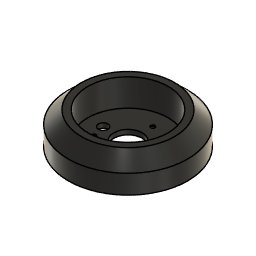
knobFlangeRev v5 (Autodesk Fusion 360 design; units mm, degrees)
Autodesk Fusion 360 part; units mm, degrees
note: some values were not read from the file. Chosen so that the rebuilt part matches the saved one: which face or edge a step refers to.
sketch "Sketch11" plane through (0, 0, 0) normal (0, 0, 1) x (1, 0, 0)
  circle A0 centre (0, 0) radius 25.25
  dimension "d97" = 50.5
  constraint coincident A0.centre origin
  measures "d97" diameter of A0
extrude "Extrude11" add sketch "Sketch11" along normal blind 17
chamfer "Chamfer8" distance 9 distance2 9 1 edges at (-23.5413, -9.1308, 17) measured on face at (8.0427, 2.4809, 17)
sketch "Sketch12" plane through (0, 0, 17) normal (0, 0, 1) x (-1, 0, 0)
  circle A0 centre (0, 0) radius 16.25
  circle A1 centre (0, 0) radius 17
  constraint coincident A0.centre A1.centre
extrude "Extrude12" cut sketch "Sketch12" against normal blind 15 contours A0 | A1
sketch "Sketch13" plane through (0, 0, 0) normal (0, 0, -1) x (1, 0, 0)
  circle A0 centre (0, 0) radius 25.25
  line L0 (0, 0) -> (0, -10.5)
  dimension "d105" = 10.5
  constraint coincident A0.centre L0.start
  constraint vertical L0
  measures "d105" distance of A0.centre L0.end
hole "Hole4" at (0, 10.5, 0) direction (0, 0, 1) diameter 1.8 depth 10 tip angle 180 counterbore diameter 3.5 counterbore depth 1.6
pattern_circular "C-Pattern9" count 3 over 360 about axis through (0, 0, 0) along (0, 0, 1) of "Hole4"
sketch "Sketch14" plane through (0, 0, 0) normal (0, 0, -1) x (1, 0, 0)
  circle A0 centre (0, 0) radius 25.25
  circle A1 centre (0, 0) radius 6
  circle A2 centre (9.0933, 5.25) radius 1.75
  circle A3 centre (-9.0933, 5.25) radius 1.75
  circle A4 centre (0, -10.5) radius 1.75
  dimension "d113" = 12
  constraint concentric A0 A1
  measures "d113" diameter of A1
extrude "Extrude13" cut sketch "Sketch14" against normal blind 20 contours A1
sketch "Sketch15" plane through (0, 0, 0) normal (0, 0, -1) x (1, 0, 0)
  circle A0 centre (0, 0) radius 6
  circle A1 centre (0, 0) radius 25.25
  circle A2 centre (0, 0) radius 23
  circle A3 centre (0, 0) radius 24.25
  circle A4 centre (9.0933, 5.25) radius 1.75
  circle A5 centre (-9.0933, 5.25) radius 1.75
  circle A6 centre (0, -10.5) radius 1.75
  dimension "d116" = 46
  dimension "d117" = 48.5
  constraint concentric A0 A2
  constraint coincident A0.centre A1.centre
  measures "d116" diameter of A2
  measures "d117" diameter of A3
extrude "Extrude14" cut sketch "Sketch15" against normal blind 2 contours A3
sketch "Sketch16" plane through (0, 0, 0) normal (0, 0, -1) x (1, 0, 0)
  circle A0 centre (0, 0) radius 23
  circle A1 centre (0, 0) radius 6
  line L0 (0, 0) -> (-10.5, 0)
  circle A2 centre (9.0933, 5.25) radius 1.75
  circle A3 centre (-9.0933, 5.25) radius 1.75
  circle A4 centre (0, -10.5) radius 1.75
  dimension "d126" = 10.5
  constraint coincident A0.centre A1.centre
  constraint horizontal L0
  measures "d126" distance of A0.centre L0.end
sketch "Sketch17" plane through (0, 0, 0) normal (0, 0, -1) x (1, 0, 0)
  circle A0 centre (0, 0) radius 23
  circle A1 centre (0, 0) radius 6
  circle A2 centre (9.0933, 5.25) radius 1.75
  circle A3 centre (-9.0933, 5.25) radius 1.75
  circle A4 centre (0, -10.5) radius 1.75
hole "Hole5" at (-10.5, 0, 0) direction (0, 0, 1) diameter 4 depth 10 tip angle 180
pattern_circular "C-Pattern11" count 2 over 360 about axis through (0, 0, 0) along (0, 0, -1) of "Hole5"
sketch "Sketch18" plane through (0, 0, 17) normal (0, 0, 1) x (-1, 0, 0)
  circle A0 centre (0, 0) radius 17
  circle A1 centre (0, 0) radius 20.25
  circle A2 centre (0, 0) radius 26
  constraint coincident A0.centre A1.centre
extrude "Extrude16" cut sketch "Sketch18" against normal blind 2 contours A1 | A2
sketch "Sketch19" plane through (0, 0, 0) normal (0, 0, 1) x (1, 0, 0)
sketch "Sketch20" plane through (0, 0, 2) normal (0, 0, -1) x (1, 0, 0)
  circle A0 centre (10.5, 0) radius 2
  circle A1 centre (-10.5, 0) radius 2
  circle A2 centre (0, 0) radius 23
  circle A3 centre (0, 0) radius 6
  circle A4 centre (9.0933, 5.25) radius 1.8
  circle A5 centre (-9.0933, 5.25) radius 1.8
  circle A6 centre (0, -10.5) radius 1.8
  line L0 (0, 0) -> (-4, 0)
  line L1 (-4, 0) -> (4, 0)
  line L2 (4, 0) -> (4, -24)
  line L3 (-4, 0) -> (-4, -24)
  circle A7 centre (0, 0) radius 23
  circle A8 centre (0, 0) radius 24.25
  line L4 (0, 0) -> (0, -2)
  line L5 (0, -2) -> (0, 2)
  line L6 (0, 2) -> (-24.1674, 2)
  line L7 (0, -2) -> (-24.1674, -2)
  dimension "d134" = 8
  dimension "d135" = 2
  constraint coincident A2.centre A3.centre
  constraint horizontal L0
  constraint parallel L0 L1
  constraint perpendicular L1 L2
  constraint perpendicular L1 L3
  constraint perpendicular L0 L4
  constraint perpendicular L1 L5
  constraint coincident A8 L6.end
  constraint perpendicular L5 L6
  constraint coincident A8 L7.end
  constraint perpendicular L4 L7
  measures "d134" distance of L0.end L1.end
  measures "d135" distance of A2.centre L4.end
extrude "Extrude17" add sketch "Sketch20" along normal blind 2 contours A2 A7 A8 L6 L7 | A2 L2 L3 A7 A8
pattern_circular "C-Pattern12" count 2 over 360 about axis through (0, 0, 0) along (0, 0, -1) of "Extrude17"
sketch "Sketch21" plane through (0, 0, 15) normal (0, 0, 1) x (-1, 0, 0)
  circle A0 centre (0, 0) radius 18.25
  circle A1 centre (0, 0) radius 17
  circle A2 centre (0, 0) radius 25.25
  dimension "d140" = 50.5
  constraint concentric A0 A2
  measures "d140" diameter of A2
extrude "Extrude18" cut sketch "Sketch21" against normal blind 1.5 contours A0 | A2
